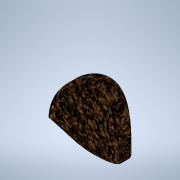
# Autodesk Inventor part: Obstacle stone
Saved by Autodesk Inventor 2021 (Build 250183000, 183)
## iProperties
Created: 2021-07-08
Part Number: Obstacle stone
Material: Generic
Document SubType Name: Modeling
Designer: shifa
Density: 1 g/cm^3
Appearance: Default
Author: shifa
Autodesk Inventor part; units mm, degrees
ref_plane "YZ Plane" through (0, 0, 0) normal (1, 0, 0) x (0, 1, 0)
ref_plane "XZ Plane" through (0, 0, 0) normal (0, 1, 0) x (-1, 0, 0)
ref_plane "XY Plane" through (0, 0, 0) normal (0, 0, 1) x (1, 0, 0)
sketch "Sketch1" plane through (0, 0, 0) normal (0, 0, 1) x (1, 0, 0)
  line L0 (0, 0) -> (0, 25.2167) construction
  line L1 (0, 25.2167) -> (58.1853, 71.3414) construction
  line L2 (58.1853, 71.3414) -> (58.1853, 0) construction
  line L3 (58.1853, 0) -> (58.1853, 0) construction
  line L4 (58.1853, 0) -> (58.1853, -8.613) construction
  line L5 (58.1853, -8.613) -> (22.8762, -8.613) construction
  line L6 (22.8762, -8.613) -> (18.6034, -4.5921) construction
  line L7 (18.6034, -4.5921) -> (0, 0) construction
  spline S0 degree 4 poles (0, 0) (0, 25.2167) (58.1853, 71.3414) (58.1853, 0) (58.1853, 0) (58.1853, -8.613) (22.8762, -8.613) (18.6034, -4.5921) (0, 0) knots 1 1 1 1 1 2 3 4 5 6 6 6 6 6
  constraints: 2 horizontal, 2 vertical, 2 other
extrude "Extrusion1" add sketch "Sketch1" along normal blind 10
fillet "Fillet2" radius 2 2 edges at (58.0627, -1.4794, 10) (58.0627, -1.4794, 0)
body "Solid1"
